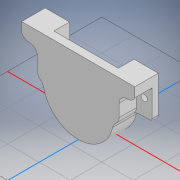
# Autodesk Inventor part: 000.002.002 - Крышка мотора задняя
Saved by Autodesk Inventor 2022 (Build 260153000, 153)
## iProperties
Created: 2022-11-07
Part Number: 000.002.002 - Крышка мотора задняя
Material: Типовые
Document SubType Name: Modeling
Designer: Petrov Ivan
Density: 1 g/cm^3
Appearance: По умолчанию
Author: Petrov Ivan
Autodesk Inventor part; units mm, degrees
ref_plane "YZ Plane" through (0, 0, 0) normal (1, 0, 0) x (0, 1, 0)
ref_plane "XZ Plane" through (0, 0, 0) normal (0, 1, 0) x (-1, 0, 0)
ref_plane "XY Plane" through (0, 0, 0) normal (0, 0, 1) x (1, 0, 0)
sketch "Эскиз3" plane through (0, 0, 0) normal (0, 0, 1) x (1, 0, 0)
  line L0 (36, 19) -> (-36, 19)
  line L1 (-36, 19) -> (-36, 1.5)
  arc A0 (-36, 1.5) -> (-34.5, 0) centre (-34.5, 1.5) ccw
  line L2 (-34.5, 0) -> (-28.1425, 0)
  arc A1 (-21.9482, -4.9523) -> (-28.1425, 0) centre (-28.1425, -6.35) ccw
  arc A2 (-21.9482, -4.9523) -> (21.9482, -4.9523) centre (0, 0) ccw
  arc A3 (28.1425, 0) -> (21.9482, -4.9523) centre (28.1425, -6.35) ccw
  line L3 (34.5, 0) -> (28.1425, 0)
  arc A4 (34.5, 0) -> (36, 1.5) centre (34.5, 1.5) ccw
  line L4 (36, 19) -> (36, 1.5)
  circle A5 centre (0, 0) radius 18.5
  line L5 (-28.1425, 0) -> (-28.1425, 19)
  line L6 (28.1425, 0) -> (28.1425, 19)
  constraints: 14 end point, 11 point on circle, 6 centre point, 2 perpendicular, 2 point on line
extrude "Выдавливание3" add sketch "Эскиз3" along normal blind 15 contours L6 A3 A2 A1 L5 L0 | A5
sketch "Эскиз4" plane through (0, 0, 0) normal (0, 0, -1) x (-1, 0, 0)
  line L0 (36, 19) -> (-36, 19)
  line L1 (-36, 19) -> (-36, 1.5)
  arc A0 (-36, 1.5) -> (-34.5, 0) centre (-34.5, 1.5) ccw
  line L2 (-34.5, 0) -> (-28.1425, 0)
  arc A1 (-21.9482, -4.9523) -> (-28.1425, 0) centre (-28.1425, -6.35) ccw
  arc A2 (-21.9482, -4.9523) -> (21.9482, -4.9523) centre (0, 0) ccw
  arc A3 (28.1425, 0) -> (21.9482, -4.9523) centre (28.1425, -6.35) ccw
  line L3 (34.5, 0) -> (28.1425, 0)
  arc A4 (34.5, 0) -> (36, 1.5) centre (34.5, 1.5) ccw
  line L4 (36, 19) -> (36, 1.5)
  circle A5 centre (0, 0) radius 18.5
  line L5 (-28.1425, 0) -> (-28.1425, 19)
  line L6 (28.1425, 0) -> (28.1425, 19)
  line L7 (-18.5, 0) -> (-18.5, 19)
  line L8 (-28.1425, 19) -> (28.1425, 19) projected
  line L9 (18.5, 0) -> (18.5, 19)
  constraints: 18 end point, 13 point on circle, 6 centre point, 4 point on line, 3 perpendicular, 1 tangent, 1 vertical
extrude "Выдавливание4" cut sketch "Эскиз4" against normal blind 10 contours L9 A5 L7 L0 | A5
offset faces "Размер1" outward -2 faces at (18.5, 12.6667, 6.6667) (-18.44, -1.4886, 6.6667) (-18.5, 6.3333, 6.6667)
offset faces "Размер2" outward 5.5 faces at (6.8333, 19, 13.3333)
sketch "Эскиз6" plane through (0, 0, 15) normal (0, 0, 1) x (1, 0, 0)
  line L0 (-28.1425, 24.5) -> (-36.0005, 24.5)
  line L1 (-36.0005, 24.5) -> (-36.0005, 0)
  line L2 (-36.0005, 0) -> (-28.1425, 0)
  line L3 (-28.1425, 0) -> (-28.1425, 24.5)
  point P0 (0, 0)
  dimension "d13" = 7.858
  constraints: 8 end point, 2 parallel, 1 horizontal, 1 perpendicular
  measures "d13" distance of L2.end L1.end
extrude "Выдавливание6" add sketch "Эскиз6" against normal up to surface (15 mm away)
mirror "Зеркальное отражение1" about plane through (0, 0, 0) normal (1, 0, 0) of "Выдавливание6"
sketch "Эскиз5" plane through (0, 0, 15) normal (0, 0, 1) x (1, 0, 0)
  circle A0 centre (-31, 10.4284) radius 2 projected
  circle A1 centre (31, 10.4284) radius 2 projected
  point P0 (0, 0)
extrude "Выдавливание5" cut sketch "Эскиз5" against normal through all
sketch "Эскиз7" plane through (0, 0, 15) normal (0, 0, 1) x (1, 0, 0)
  circle A0 centre (-31, 10.4284) radius 2 projected
  circle A1 centre (-31, 10.4284) radius 5.0005
  line L0 (-36.0005, 24.5) -> (-36.0005, 0) projected
  circle A2 centre (31, 10.4284) radius 2 projected
  circle A3 centre (31, 10.4284) radius 5.0005
  line L1 (36.0005, 24.5) -> (36.0005, 0) projected
  arc A4 (-36.0005, 18.4308) -> (-33.5949, 14.7029) centre (-27.8544, 21.0474) ccw
  line L2 (-31, 10.4284) -> (-36.0005, 10.4284) construction
  line L3 (-25.9995, 10.4284) -> (-25.9995, -0.3725)
  arc A5 (-21.9482, -4.9523) -> (-28.1425, 0) centre (-28.1425, -6.35) ccw projected
  line L4 (-36.0005, 0) -> (-28.1425, 0) projected
  point P0 (0, 0)
  point P1 (-33.5949, 6.1538)
  point P2 (-36.0005, 2.4259)
  constraints: 7 point on circle, 4 end point, 3 centre point, 3 point on line, 2 coincident, 2 tangent, 1 vertical
extrude "Выдавливание7" cut sketch "Эскиз7" against normal blind 11 contours A1 | L3 A5 L4 L0 A1 | A1 L0 A4
mirror "Зеркальное отражение2" about plane through (0, 0, 0) normal (1, 0, 0) of "Выдавливание7"
fillet "Сопряжение6" radius 5 4 edges at (-33.5949, 14.7029, 9.5) (33.5949, 14.7029, 9.5) (25.9995, -0.3725, 9.5) (-25.9995, -0.3725, 9.5)
fillet "Сопряжение7" radius 1.5 2 edges at (-36.0005, 0, 2) (36.0005, 0, 2)
